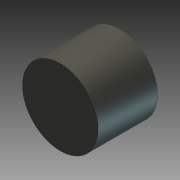
# Autodesk Inventor part: Motor - DT750
Saved by Autodesk Inventor 2012 (Build 160160000, 160)
## iProperties
Created: 2013-03-14
Part Number: Motor - DT750
Material: Default
Document SubType Name: Modeling
Designer: fixer
Mass: 86 g
Surface Area: 66.48 cm^2
Volume: 41.1852 cm^3
Density: 2.08813 g/cm^3
Author: fixer
Autodesk Inventor part; units mm, degrees
ref_plane "YZ Plane" through (0, 0, 0) normal (1, 0, 0) x (0, 1, 0)
ref_plane "XZ Plane" through (0, 0, 0) normal (0, 1, 0) x (-1, 0, 0)
ref_plane "XY Plane" through (0, 0, 0) normal (0, 0, 1) x (1, 0, 0)
sketch "Sketch1" plane through (0, 0, 0) normal (0, 0, 1) x (1, 0, 0)
  circle A0 centre (0, 0) radius 20.32
  dimension "d0" = 40.64
  dimension "d0" = 40.64
  constraints: 1 centre point, 1 coincident
  measures "d0" diameter of A0
extrude "Extrusion1" add sketch "Sketch1" along normal blind 31.75
body "Solid1"
